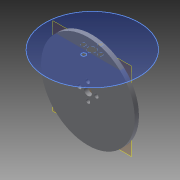
# Autodesk Inventor part: gearGuideRings
Saved by Autodesk Inventor 2013 (Build 170138000, 138)
## iProperties
Created: 2013-02-22
Part Number: gearGuideRings
Material: Generic
Document SubType Name: Modeling
Designer: Nano
Density: 1 g/cm^3
Author: Nano
Autodesk Inventor part; units mm, degrees
ref_plane "YZ Plane" through (0, 0, 0) normal (1, 0, 0) x (0, 1, 0)
ref_plane "XZ Plane" through (0, 0, 0) normal (0, 1, 0) x (-1, 0, 0)
ref_plane "XY Plane" through (0, 0, 0) normal (0, 0, 1) x (1, 0, 0)
ref_plane "Work Plane1" through (0, 0, 0) normal (0, 0, 1) x (1, 0, 0)
sketch "Sketch1" plane through (0, 0, 0) normal (0, 0, 1) x (1, 0, 0)
  circle A0 centre (-0.1312, 6.3486) radius 1.5875
  circle A1 centre (6.3486, 0.1312) radius 1.5875
  circle A2 centre (0.1312, -6.3486) radius 1.5875
  circle A3 centre (-6.3486, -0.1312) radius 1.5875
  arc A4 (-1.8, 2.4) -> (1.8, 2.4) centre (0, 0) ccw
  arc A5 (-10.2062, 24.6399) -> (-9.5905, 18.6316) centre (10.2722, 23.7027) ccw
  arc A6 (-9.5905, 18.6316) -> (-11.0963, 17.7759) centre (0, 0) ccw
  arc A7 (-11.0963, 17.7759) -> (-15.9426, 21.3804) centre (-25.6201, 3.3086) ccw
  arc A8 (-15.9426, 21.3804) -> (-17.6537, 19.9909) centre (0, 0) ccw
  arc A9 (-17.6537, 19.9909) -> (-15.1205, 14.508) centre (2.0194, 25.7538) ccw
  arc A10 (-15.1205, 14.508) -> (-16.2669, 13.2098) centre (0, 0) ccw
  arc A11 (-16.2669, 13.2098) -> (-22.021, 15.0454) centre (-25.3062, -5.1895) ccw
  arc A12 (-22.021, 15.0454) -> (-23.1882, 13.1756) centre (0, 0) ccw
  arc A13 (-23.1882, 13.1756) -> (-19.012, 8.8123) centre (-6.4522, 25.0141) ccw
  arc A14 (-19.012, 8.8123) -> (-19.6747, 7.2122) centre (0, 0) ccw
  arc A15 (-19.6747, 7.2122) -> (-25.7131, 7.08) centre (-22.2501, -13.1252) ccw
  arc A16 (-25.7131, 7.08) -> (-26.2099, 4.9325) centre (0, 0) ccw
  arc A17 (-26.2099, 4.9325) -> (-20.8432, 2.1617) centre (-14.2247, 21.5637) ccw
  arc A18 (-20.8432, 2.1617) -> (-20.9505, 0.4331) centre (0, 0) ccw
  arc A19 (-20.9505, 0.4331) -> (-26.6187, -1.6526) centre (-16.7827, -19.6386) ccw
  arc A20 (-26.6187, -1.6526) -> (-26.3914, -3.8451) centre (0, 0) ccw
  arc A21 (-26.3914, -3.8451) -> (-20.4158, -4.7232) centre (-20.4557, 15.7766) ccw
  arc A22 (-20.4158, -4.7232) -> (-19.956, -6.393) centre (0, 0) ccw
  arc A23 (-19.956, -6.393) -> (-24.6399, -10.2062) centre (-9.4967, -24.0239) ccw
  arc A24 (-24.6399, -10.2062) -> (-23.7129, -12.2061) centre (0, 0) ccw
  arc A25 (-23.7129, -12.2061) -> (-17.7759, -11.0963) centre (-24.47, 8.2798) ccw
  arc A26 (-17.7759, -11.0963) -> (-16.7989, -12.5263) centre (0, 0) ccw
  arc A27 (-16.7989, -12.5263) -> (-19.9909, -17.6537) centre (-1.1816, -25.8058) ccw
  arc A28 (-19.9909, -17.6537) -> (-18.4648, -19.2443) centre (0, 0) ccw
  arc A29 (-18.4648, -19.2443) -> (-13.2098, -16.2669) centre (-25.8326, -0.1142) ccw
  arc A30 (-13.2098, -16.2669) -> (-11.8214, -17.3022) centre (0, 0) ccw
  arc A31 (-11.8214, -17.3022) -> (-13.1756, -23.1882) centre (7.2615, -24.7913) ccw
  arc A32 (-13.1756, -23.1882) -> (-11.2157, -24.197) centre (0, 0) ccw
  arc A33 (-11.2157, -24.197) -> (-7.2122, -19.6747) centre (-24.3958, -8.4958) ccw
  arc A34 (-7.2122, -19.6747) -> (-5.5629, -20.2031) centre (0, 0) ccw
  arc A35 (-5.5629, -20.2031) -> (-4.9325, -26.2099) centre (14.9178, -21.0902) ccw
  arc A36 (-4.9325, -26.2099) -> (-2.7512, -26.5277) centre (0, 0) ccw
  arc A37 (-2.7512, -26.5277) -> (-0.4331, -20.9505) centre (-20.3154, -15.9568) ccw
  arc A38 (-0.4331, -20.9505) -> (1.2985, -20.9147) centre (0, 0) ccw
  arc A39 (1.2985, -20.9147) -> (3.8451, -26.3914) centre (20.9575, -15.1037) ccw
  arc A40 (3.8451, -26.3914) -> (6.0114, -25.9837) centre (0, 0) ccw
  arc A41 (6.0114, -25.9837) -> (6.393, -19.956) centre (-14.0335, -21.6886) ccw
  arc A42 (6.393, -19.956) -> (8.0191, -19.3599) centre (0, 0) ccw
  arc A43 (8.0191, -19.3599) -> (12.2061, -23.7129) centre (24.7261, -7.4804) ccw
  arc A44 (12.2061, -23.7129) -> (14.1226, -22.6239) centre (0, 0) ccw
  arc A45 (14.1226, -22.6239) -> (12.5263, -16.7989) centre (-6.2308, -25.0702) ccw
  arc A46 (12.5263, -16.7989) -> (13.8708, -15.7071) centre (0, 0) ccw
  arc A47 (13.8708, -15.7071) -> (19.2443, -18.4648) centre (25.8152, 0.9534) ccw
  arc A48 (19.2443, -18.4648) -> (20.7033, -16.8125) centre (0, 0) ccw
  arc A49 (20.7033, -16.8125) -> (17.3022, -11.8214) centre (2.2471, -25.7349) ccw
  arc A50 (17.3022, -11.8214) -> (18.2193, -10.3522) centre (0, 0) ccw
  arc A51 (18.2193, -10.3522) -> (24.197, -11.2157) centre (24.1069, 9.284) ccw
  arc A52 (24.197, -11.2157) -> (25.0406, -9.1792) centre (0, 0) ccw
  arc A53 (25.0406, -9.1792) -> (20.2031, -5.5629) centre (10.4814, -23.6109) ccw
  arc A54 (20.2031, -5.5629) -> (20.5935, -3.8755) centre (0, 0) ccw
  arc A55 (20.5935, -3.8755) -> (26.5277, -2.7512) centre (19.7863, 16.6084) ccw
  arc A56 (26.5277, -2.7512) -> (26.6643, -0.5512) centre (0, 0) ccw
  arc A57 (26.6643, -0.5512) -> (20.9147, 1.2985) centre (17.58, -18.9283) ccw
  arc A58 (20.9147, 1.2985) -> (20.7361, 3.0212) centre (0, 0) ccw
  arc A59 (20.7361, 3.0212) -> (25.9837, 6.0114) centre (13.3214, 22.1331) ccw
  arc A60 (25.9837, 6.0114) -> (25.3985, 8.1366) centre (0, 0) ccw
  arc A61 (25.3985, 8.1366) -> (19.3599, 8.0191) centre (22.7734, -12.1945) ccw
  arc A62 (19.3599, 8.0191) -> (18.6316, 9.5905) centre (0, 0) ccw
  arc A63 (18.6316, 9.5905) -> (22.6239, 14.1226) centre (5.413, 25.2594) ccw
  arc A64 (22.6239, 14.1226) -> (21.3804, 15.9426) centre (0, 0) ccw
  arc A65 (21.3804, 15.9426) -> (15.7071, 13.8708) centre (25.4991, -4.1393) ccw
  arc A66 (15.7071, 13.8708) -> (14.508, 15.1205) centre (0, 0) ccw
  arc A67 (14.508, 15.1205) -> (16.8125, 20.7033) centre (-3.082, 25.6483) ccw
  arc A68 (16.8125, 20.7033) -> (15.0454, 22.021) centre (0, 0) ccw
  arc A69 (15.0454, 22.021) -> (10.3522, 18.2193) centre (25.4615, 4.3646) ccw
  arc A70 (10.3522, 18.2193) -> (8.8123, 19.012) centre (0, 0) ccw
  arc A71 (8.8123, 19.012) -> (9.1792, 25.0406) centre (-11.243, 23.2579) ccw
  arc A72 (9.1792, 25.0406) -> (7.08, 25.7131) centre (0, 0) ccw
  arc A73 (7.08, 25.7131) -> (3.8755, 20.5935) centre (22.6647, 12.3954) ccw
  arc A74 (3.8755, 20.5935) -> (2.1617, 20.8432) centre (0, 0) ccw
  arc A75 (2.1617, 20.8432) -> (0.5512, 26.6643) centre (-18.1856, 18.3472) ccw
  arc A76 (0.5512, 26.6643) -> (-1.6526, 26.6187) centre (0, 0) ccw
  arc A77 (-1.6526, 26.6187) -> (-3.0212, 20.7361) centre (17.4119, 19.083) ccw
  arc A78 (-3.0212, 20.7361) -> (-4.7232, 20.4158) centre (0, 0) ccw
  arc A79 (-4.7232, 20.4158) -> (-8.1366, 25.3985) centre (-23.1576, 11.4482) ccw
  arc A80 (-8.1366, 25.3985) -> (-10.2062, 24.6399) centre (0, 0) ccw
  circle A81 centre (0, 0) radius 34.925
  line L0 (-3.1504, 2.4) -> (-1.8, 2.4)
  line L1 (1.8, 2.4) -> (3.3261, 2.4)
  line L2 (-1.8, 2.4) -> (1.8, 2.4)
  point P0 (0.0879, -3)
  dimension "d0" = 69.85
  dimension "d3" = 6
  dimension "d4" = 5.4
  constraints: 154 point on circle, 82 centre point, 6 end point, 1 other
  measures "d0" diameter of A81
  measures "d3" diameter of A4
  measures "d4" distance from line of point (0.088, -3) L0
extrude "Extrusion1" add sketch "Sketch1" along normal blind 3.175 contours A80 A79 A78 A77 A76 A75 A74 A73 A72 A71 A70 A69 A68 A67 A66 A65 A64 A63 A62 A61 A60 A59 A58 A57 A56 A55 A54 A53 A52 A51 A50 A49 A48 A47 A46 A45 A44 A43 A42 A41 A40 A39 A38 A37 A36 A35 A34 A33 A32 A31 A30 A29 A28 A27 A26 A25 A24 A23 A22 A21 A20 A19 A18 A17 A16 A15 A14 A13 A12 A11 A10 A9 A8 A7 A6 A5 | A81
body "Solid1"
